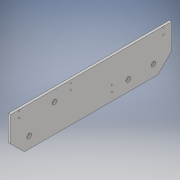
# Autodesk Inventor part: DriveTrain3.0
Saved by Autodesk Inventor 2017 (Build 210142000, 142)
## iProperties
Created: 2017-07-22
Part Number: DriveTrain3.0
Material: Generic
Document SubType Name: Modeling
Designer: User
Density: 1 g/cm^3
Appearance: Default
Author: User
Autodesk Inventor part; units mm, degrees
ref_plane "YZ Plane" through (0, 0, 0) normal (1, 0, 0) x (0, 1, 0)
ref_plane "XZ Plane" through (0, 0, 0) normal (0, 1, 0) x (-1, 0, 0)
ref_plane "XY Plane" through (0, 0, 0) normal (0, 0, 1) x (1, 0, 0)
sketch "Sketch1" plane through (0, 0, 0) normal (1, 0, 0) x (0, 1, 0)
  line L0 (0, 0) -> (107.95, 0)
  line L1 (107.95, 0) -> (107.95, -444.5)
  line L2 (107.95, -444.5) -> (0, -444.5)
  line L3 (0, -444.5) -> (0, 0)
  circle A0 centre (31.75, -50.8) radius 6.3627
  circle A1 centre (31.75, -393.7) radius 6.3627
  circle A2 centre (92.6338, -165.5318) radius 1.5875
  circle A3 centre (76.6318, -165.5318) radius 1.5875
  circle A4 centre (15.3162, -278.9682) radius 1.5875
  circle A5 centre (31.3182, -278.9682) radius 1.5875
  dimension "d0" = 107.95
  dimension "d1" = 444.5
  dimension "d2" = 12.7254
  dimension "d3" = 31.75
  dimension "d4" = 50.8
  dimension "d5" = 50.8
  dimension "d22" = 165.5318
  dimension "d23" = 3.175
  dimension "d24" = 15.3162
  dimension "d25" = 3.175
  dimension "d26" = 16.002
  dimension "d27" = 165.5318
  dimension "d28" = 3.175
  dimension "d29" = 15.3162
  dimension "d30" = 165.5318
  dimension "d31" = 3.175
  dimension "d32" = 16.002
  dimension "d33" = 165.5318
  constraints: 8 end point, 6 centre point, 2 parallel, 1 horizontal, 1 perpendicular
  measures "d0" distance of L1.end L2.end
  measures "d1" distance of L0.end L1.end
  measures "d2" diameter of A0
  measures "d3" distance from line of L3 A0.centre
  measures "d4" distance from line of L0 A0.centre
  measures "d5" distance from line of L2 A1.centre
  measures "d22" distance from line of L0 A2.centre
  measures "d23" diameter of A2
  measures "d24" distance from line of L1 A2.centre
  measures "d25" diameter of A3
  measures "d26" distance of A2.centre A3.centre
  measures "d27" distance from line of L0 A3.centre
  measures "d28" diameter of A4
  measures "d29" distance from line of L3 A4.centre
  measures "d30" distance from line of L2 A4.centre
  measures "d31" diameter of A5
  measures "d32" distance of A5.centre A4.centre
  measures "d33" distance from line of L2 A5.centre
extrude "Extrusion1" add sketch "Sketch1" along normal blind 6.35 contours L0 L1 L2 L3 | A2 | A3 | A4 | A5
chamfer "Chamfer1" distance 38.1 angle 45 1 edges at (3.175, 0, 0)
chamfer "Chamfer2" distance 38.1 angle 45 1 edges at (3.175, 0, -444.5)
sketch "Sketch2" plane through (6.35, 0, 0) normal (1, 0, 0) x (0, 0, -1)
  line L0 (444.5, 38.1) -> (406.4, 0) projected
  line L1 (444.5, 38.1) -> (444.5, 107.95) projected
  line L2 (444.5, 107.95) -> (0, 107.95) projected
  line L3 (0, 107.95) -> (0, 38.1) projected
  line L4 (38.1, 0) -> (0, 38.1) projected
  line L5 (38.1, 0) -> (406.4, 0) projected
  circle A0 centre (393.7, 31.75) radius 6.3627 projected
  circle A1 centre (50.8, 31.75) radius 6.3627 projected
  circle A2 centre (120.4214, 77.9526) radius 6.3627
  circle A3 centre (324.0786, 29.9974) radius 6.3627
  point P0 (0, 0)
  dimension "d14" = 12.7254
  dimension "d15" = 120.4214
  dimension "d16" = 29.9974
  dimension "d17" = 12.7254
  dimension "d18" = 29.9974
  dimension "d19" = 120.4214
  constraints: 2 centre point
  measures "d14" diameter of A2
  measures "d15" distance from line of L3 A2.centre
  measures "d16" distance from line of L2 A2.centre
  measures "d17" diameter of A3
  measures "d18" distance from line of L5 A3.centre
  measures "d19" distance from line of L1 A3.centre
extrude "Extrusion2" cut sketch "Sketch2" against normal blind 25.4 contours A2 | A3
sketch "Sketch3" plane through (6.35, 0, 0) normal (1, 0, 0) x (0, 0, -1)
  circle A0 centre (120.4214, 77.9526) radius 6.3627 projected
  circle A1 centre (324.0786, 29.9974) radius 6.3627 projected
  line L0 (444.5, 38.1) -> (406.4, 0) projected
  line L1 (444.5, 38.1) -> (444.5, 107.95) projected
  line L2 (444.5, 107.95) -> (0, 107.95) projected
  line L3 (0, 107.95) -> (0, 38.1) projected
  line L4 (38.1, 0) -> (0, 38.1) projected
  line L5 (38.1, 0) -> (406.4, 0) projected
  circle A2 centre (393.7, 31.75) radius 6.3627 projected
  circle A3 centre (50.8, 31.75) radius 6.3627 projected
  circle A4 centre (165.5318, 99.949) radius 1.5875
  circle A5 centre (165.5318, 83.947) radius 1.5875
  circle A6 centre (278.9682, 22.86) radius 1.5875
  circle A7 centre (278.9682, 38.862) radius 1.5875
  point P0 (0, 0)
  dimension "d34" = 3.175
  dimension "d35" = 165.5318
  dimension "d36" = 8.001
  dimension "d37" = 3.175
  dimension "d38" = 16.002
  dimension "d39" = 3.175
  dimension "d40" = 3.175
  dimension "d41" = 22.86
  dimension "d42" = 16.002
  dimension "d43" = 165.5318
  constraints: 4 centre point
  measures "d34" diameter of A4
  measures "d35" distance from line of L3 A4.centre
  measures "d36" distance from line of L2 A4.centre
  measures "d37" diameter of A5
  measures "d38" distance of A4.centre A5.centre
  measures "d39" diameter of A6
  measures "d40" diameter of A7
  measures "d41" distance from line of L5 A6.centre
  measures "d42" distance of A7.centre A6.centre
  measures "d43" distance from line of L1 A6.centre
extrude "Extrusion3" cut sketch "Sketch3" against normal blind 25.4 contours A4 | A5 | A6 | A7
sketch "Sketch5" plane through (6.35, 0, 0) normal (1, 0, 0) x (0, 0, -1)
  circle A0 centre (278.9682, 22.86) radius 1.5875 projected
  circle A1 centre (165.5318, 99.949) radius 1.5875 projected
  circle A2 centre (165.5318, 83.947) radius 1.5875 projected
  circle A3 centre (278.9682, 38.862) radius 1.5875 projected
  circle A4 centre (120.4214, 77.9526) radius 6.3627 projected
  circle A5 centre (324.0786, 29.9974) radius 6.3627 projected
  line L0 (444.5, 38.1) -> (406.4, 0) projected
  line L1 (444.5, 38.1) -> (444.5, 107.95) projected
  line L2 (444.5, 107.95) -> (0, 107.95) projected
  line L3 (0, 107.95) -> (0, 38.1) projected
  line L4 (38.1, 0) -> (0, 38.1) projected
  line L5 (38.1, 0) -> (406.4, 0) projected
  circle A6 centre (393.7, 31.75) radius 6.3627 projected
  circle A7 centre (50.8, 31.75) radius 6.3627 projected
  circle A8 centre (23.0124, 105.5624) radius 1.9685
  circle A9 centre (23.0124, 88.1126) radius 1.9685
  circle A10 centre (421.5384, 105.5624) radius 1.9685
  circle A11 centre (421.5384, 88.1126) radius 1.9685
  point P0 (0, 0)
  dimension "d59" = 3.937
  dimension "d60" = 23.0124
  dimension "d61" = 2.3876
  dimension "d62" = 3.937
  dimension "d64" = 3.937
  dimension "d65" = 3.937
  dimension "d66" = 2.3876
  dimension "d68" = 22.9616
  dimension "d71" = 19.8374
  dimension "d72" = 19.8374
  constraints: 4 centre point
  measures "d59" diameter of A8
  measures "d60" distance from line of A8.centre L3
  measures "d61" distance from line of L2 A8.centre
  measures "d62" diameter of A9
  measures "d64" diameter of A10
  measures "d65" diameter of A11
  measures "d66" distance from line of L2 A10.centre
  measures "d68" distance from line of L1 A10.centre
  measures "d71" distance from line of A9.centre L2
  measures "d72" distance from line of L2 A11.centre
extrude "Extrusion5" cut sketch "Sketch5" against normal blind 25.4 contours A8 | A9 | A10 | A11
body "Solid1"
